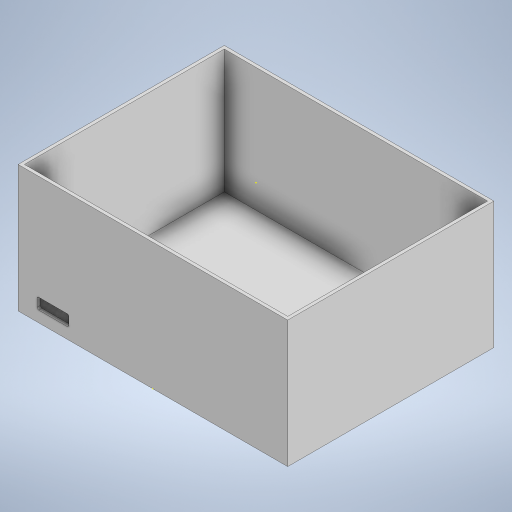
# Autodesk Inventor part: timer and thermometer
Saved by Autodesk Inventor 2024 (Build 280153000, 153)
## iProperties
Created: 2023-07-12
Part Number: timer and thermometer
Material: Generic
Document SubType Name: Modeling
Designer: thoma
Density: 1 g/cm^3
Appearance: Default
Author: thoma
Autodesk Inventor part; units mm, degrees
ref_plane "YZ Plane" through (0, 0, 0) normal (1, 0, 0) x (0, 1, 0)
ref_plane "XZ Plane" through (0, 0, 0) normal (0, 1, 0) x (-1, 0, 0)
ref_plane "XY Plane" through (0, 0, 0) normal (0, 0, 1) x (1, 0, 0)
sketch "Sketch1" plane through (0, 0, 0) normal (0, 1, 0) x (-1, 0, 0)
  line L0 (42.5, -32.5) -> (-42.5, -32.5)
  line L1 (-42.5, -32.5) -> (-42.5, 32.5)
  line L2 (-42.5, 32.5) -> (42.5, 32.5)
  line L3 (42.5, 32.5) -> (42.5, -32.5)
  point P0 (0, 0)
  point P1 (42.5, 0)
  point P2 (0, -32.5)
  dimension "d0" = 85
  dimension "d1" = 65
  constraints: 8 end point, 2 midpoint, 2 parallel, 1 horizontal, 1 horizontal alignment, 1 perpendicular, 1 vertical alignment
  measures "d0" distance of L0.start L0.end
  measures "d1" distance of L2.end L0.start
extrude "Extrusion1" add sketch "Sketch1" along normal blind 40
sketch "Sketch2" plane through (0, 40, 0) normal (0, 1, 0) x (1, 0, 0)
  point P0 (0, 0)
shell "Shell1" thickness 1 removed faces 1 at (14.1667, 40, 10.8333)
sketch "Sketch4" plane through (-42.5, 0, 32.5) normal (0, 0, 1) x (1, 0, 0)
  line L0 (6, 7) -> (16, 7)
  line L1 (16, 7) -> (16, 3.5)
  line L2 (16, 3.5) -> (6, 3.5)
  line L3 (6, 3.5) -> (6, 7)
  line L4 (0, 0) -> (0, 40) projected
  line L5 (0, 0) -> (85, 0) projected
  point P0 (42.5, 0)
  dimension "d7" = 10
  dimension "d8" = 3.5
  dimension "d9" = 6
  dimension "d10" = 3.5
  constraints: 8 end point, 2 parallel, 1 horizontal, 1 perpendicular
  measures "d7" distance of L0.start L0.end
  measures "d8" distance of L0.end L1.end
  measures "d9" distance between parallel lines of L4 L3
  measures "d10" distance between parallel lines of L5 L2
extrude "Extrusion3" cut sketch "Sketch4" against normal blind 3
sketch "Sketch5" plane through (-42.5, 0, 32.5) normal (0, 0, 1) x (1, 0, 0)
  point P0 (42.5, 0)
fillet "Fillet1" radius 0.5 4 edges at (-26.5, 7, 32) (-36.5, 7, 32) (-26.5, 3.5, 32) (-36.5, 3.5, 32)
body "Solid1"
